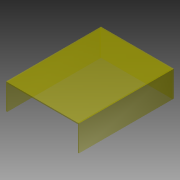
# Autodesk Inventor part: shield
Saved by Autodesk Inventor 2014 SP2 (Build 180246200, 246)
## iProperties
Created: 2016-10-02
Part Number: shield
Material: Generic
Document SubType Name: Modeling
Designer: cruiser
Density: 1 g/cm^3
Appearance: Default
Mass: 317.509 g
Surface Area: 2102.89 cm^2
Volume: 317.509 cm^3
Author: cruiser
Autodesk Inventor part; units mm, degrees
ref_plane "YZ Plane" through (0, 0, 0) normal (1, 0, 0) x (0, 1, 0)
ref_plane "XZ Plane" through (0, 0, 0) normal (0, 1, 0) x (-1, 0, 0)
ref_plane "XY Plane" through (0, 0, 0) normal (0, 0, 1) x (1, 0, 0)
sketch "Sketch1" plane through (0, 0, 0) normal (0, 0, 1) x (1, 0, 0)
  line L0 (-96.95, -128.375) -> (96.95, -128.375)
  line L1 (96.95, -128.375) -> (96.95, 128.375)
  line L2 (96.95, 128.375) -> (-96.95, 128.375)
  line L3 (-96.95, 128.375) -> (-96.95, -128.375)
  line L4 (-96.95, -128.375) -> (96.95, 128.375) construction
  line L5 (96.95, -128.375) -> (-96.95, 128.375) construction
  point P0 (0, 0)
  dimension "d0" = 193.9
  dimension "d1" = 256.75
  constraints: 12 end point, 2 midpoint, 2 parallel, 1 horizontal, 1 perpendicular
  measures "d0" distance of L2.end L1.end
  measures "d1" distance of L1.end L0.end
extrude "Extrusion1" add sketch "Sketch1" against normal blind 3.15
sketch "Sketch2" plane through (96.95, -128.375, 0) normal (1, 0, 0) x (0, 0, -1)
  line L0 (0, 256.75) -> (71, 256.75)
  line L1 (71, 256.75) -> (71, 0)
  line L2 (71, 0) -> (0, 0)
  line L3 (0, 0) -> (0, 256.75)
  point P0 (0, 128.375)
  dimension "d4" = 71
  dimension "d5" = 256.75
  constraints: 8 end point, 2 parallel, 1 horizontal, 1 perpendicular
  measures "d4" distance of L1.end L2.end
  measures "d5" distance of L0.end L1.end
extrude "Extrusion2" add sketch "Sketch2" along normal blind 3.15 separate body
mirror "Mirror1" about plane through (0, 0, 0) normal (1, 0, 0) bodies 2
sketch "Sketch3" plane through (-96.95, 128.375, 0) normal (0, 1, 0) x (1, 0, 0)
  line L0 (193.9, 0) -> (0, 0) projected
  line L1 (-3.15, 0) -> (197.05, 0)
  line L2 (197.05, 0) -> (197.05, 71)
  line L3 (197.05, 71) -> (-3.15, 71)
  line L4 (-3.15, 71) -> (-3.15, 0)
  line L5 (-3.15, 71) -> (-3.15, 0) projected
  point P0 (96.95, 0)
  dimension "d8" = 200.2
  dimension "d9" = 71
  constraints: 8 end point, 2 collinear, 2 parallel, 1 horizontal, 1 perpendicular
  measures "d8" distance of L3.end L2.end
  measures "d9" distance of L2.end L1.end
extrude "Extrusion3" add sketch "Sketch3" along normal blind 3.15 separate body
equation "\"d0\" = shield_x - 2 * shield_t"
equation "\"d1\" = shield_z - shield_t"
equation "\"d2\" = shield_t"
equation "\"d4\" = shield_y"
equation "\"d5\" = shield_z - shield_t"
equation "\"d6\" = shield_t"
equation "\"d8\" = shield_x"
equation "\"d9\" = shield_y"
equation "\"d10\" = shield_t"
equation "\"laserresin\" = 5"
equation "\"st1_thickness\" = 0.91186"
equation "\"st2_thickness\" = 1.5875"
equation "\"al1_thickness\" = 0.79375"
equation "\"al2_thickness\" = 1.5875"
equation "\"bend_factor\" = 2.26205"
equation "\"st1_bend\" = 2.06267"
equation "\"st2_bend\" = 3.591"
equation "\"st3_bend\" = 113.10236"
equation "\"al1_bend\" = 1.7955"
equation "\"al2_bend\" = 3.591"
equation "\"al3_bend\" = 113.10236"
equation "\"acrylic1_thickness\" = 5.88"
equation "\"acrylic2_thickness\" = 3.15"
equation "\"acrylic3_thickness\" = 3.15"
equation "\"corner_small_r\" = 1"
equation "\"corner_big_r\" = 5"
equation "\"linear_bearing_spacing\" = 208"
equation "\"galvo_y_out_offset\" = 27"
equation "\"galvo_y_in_offset\" = 17.5"
equation "\"laser_diameter\" = 13"
equation "\"nema17_x\" = 43"
equation "\"nema17_shaft\" = 24"
equation "\"lmk8uu_x\" = 25"
equation "\"lmk8uu_shaft\" = 15"
equation "\"lmk8uu_z\" = 24"
equation "\"shf8_y\" = 43"
equation "\"acme_nut_d\" = 19.1"
equation "\"acme_nut_upper_d\" = 12.7"
equation "\"handle_spacing\" = 50.8"
equation "\"handle_d\" = 4.7625"
equation "\"handle_hole_d\" = 2.845"
equation "\"handle_projection\" = 20.6375"
equation "\"switch_spacing\" = 19"
equation "\"laser_body_diameter\" = 12"
equation "\"m3_diameter\" = 3"
equation "\"m3_head\" = 6"
equation "\"m4_diameter\" = 4"
equation "\"m5_diameter\" = 5"
equation "\"m5_head\" = 10.3"
equation "\"rivet1_diameter\" = 3.26"
equation "\"rivet2_diameter\" = 3.26"
equation "\"brass_insert_drill\" = 4"
equation "\"m5_brass_insert_drill\" = 6.7"
equation "\"m3_press_nut_drill\" = 4.5"
equation "\"m5_press_nut_drill\" = 6.5"
equation "\"platform_t\" = 1.5875"
equation "\"platform_z\" = 65"
equation "\"platform_fold_x\" = 15"
equation "\"platform_crane_gap\" = 0.1"
equation "\"platform_gap\" = 0.1"
equation "\"platform_upper_y\" = 46.625"
equation "\"crane_t\" = 1.5875"
equation "\"crane_x\" = 233"
equation "\"crane_gap\" = 0.1"
equation "\"tray_t\" = 5.88"
equation "\"tray_to_platform_oversize\" = 0"
equation "\"reservoir_t\" = 0.91186"
equation "\"reservoir_z\" = 35"
equation "\"reservoir_flap_y\" = 20.91186"
equation "\"frame_front_t\" = 0.91186"
equation "\"frame_front_y\" = 56"
equation "\"frame_front_fold\" = 15"
equation "\"frame_gap\" = 0.1"
equation "\"frame_back_t\" = 0.91186"
equation "\"frame_back_x\" = 277.97628"
equation "\"frame_back_y\" = 53.97628"
equation "\"frame_back_z\" = 497.97628"
equation "\"drawer_t\" = 0.91186"
equation "\"drawer_gap\" = 0.1"
equation "\"drawer_reservoir_overlap_x\" = 24.08814"
equation "\"drawer_x\" = 202.02372"
equation "\"drawer_y\" = 73"
equation "\"drawer_seal_y\" = 101"
equation "\"drawer_window_gap\" = 6"
equation "\"foot_t\" = 0.91186"
equation "\"foot_x\" = 198"
equation "\"foot_y\" = 196"
equation "\"laser_holder_t\" = 0.91186"
equation "\"laser_holder_z\" = 75"
equation "\"laser_offset_x\" = 59"
equation "\"laser_offset_y\" = 8.5"
equation "\"subframe_t\" = 0.79375"
equation "\"subframe_x\" = 66"
equation "\"subframe_y\" = 55"
equation "\"shield_x\" = 200.2"
equation "\"shield_y\" = 71"
equation "\"shield_z\" = 259.9"
equation "\"shield_t\" = 3.15"
equation "\"magnet_w\" = 12.8"
equation "\"magnet_t\" = 1.6"
equation "\"sae_4_40_diameter\" = 2.845"
body "Solid1"
body "Solid2"
body "Solid3"
body "Solid4"
